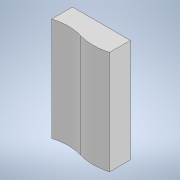
# Autodesk Inventor part: Ground2
Saved by Autodesk Inventor 2021 (Build 250183000, 183)
## iProperties
Created: 2022-07-02
Part Number: Ground2
Material: 一般
Document SubType Name: Modeling
Designer: tazak
Density: 1 g/cm^3
Appearance: 既定
Author: tazak
Autodesk Inventor part; units mm, degrees
ref_plane "YZ Plane" through (0, 0, 0) normal (1, 0, 0) x (0, 1, 0)
ref_plane "XZ Plane" through (0, 0, 0) normal (0, 1, 0) x (-1, 0, 0)
ref_plane "XY Plane" through (0, 0, 0) normal (0, 0, 1) x (1, 0, 0)
sketch "スケッチ1" plane through (0, 0, 0) normal (0, 0, 1) x (1, 0, 0)
  line L0 (2000, 2500) -> (4800, 2500)
  line L1 (4800, 2500) -> (4800, -2500)
  line L2 (4800, -2500) -> (2000, -2500)
  line L3 (2000, -2500) -> (2000, 2500)
  point P0 (0, 0)
  point P1 (2000, 0)
  dimension "d2" = 5000
  dimension "d5" = 2000
  dimension "d6" = 2800
  constraints: 8 end point, 2 parallel, 1 horizontal, 1 horizontal alignment, 1 midpoint, 1 perpendicular
  measures "d2" distance of L2.end L0.start
  measures "d5" distance from line of L3 point (0, 0)
  measures "d6" distance of L0.start L0.end
extrude "押し出し1" add sketch "スケッチ1" against normal blind 1000
sketch "スケッチ2" plane through (2000, -2500, 0) normal (0, -1, 0) x (1, 0, 0)
  circle A0 centre (700, 2400) radius 2500
  line L0 (0, 0) -> (2800, 0) projected
  point P0 (-2000, 0)
  point P1 (1400, 0)
  dimension "d7" = 5000
  constraints: 2 point on circle, 1 centre point, 1 midpoint
  measures "d7" diameter of A0
extrude "押し出し2" cut sketch "スケッチ2" against normal through all
sketch "スケッチ3" plane through (2000, -2500, -1000) normal (0, -1, 0) x (1, 0, 0)
  line L0 (2800, 1000) -> (1400, 1000) projected
  circle A0 centre (2100, -1400) radius 2500
  point P0 (-2000, 1000)
  dimension "d10" = 5000
  constraints: 2 point on circle, 1 centre point
  measures "d10" diameter of A0
extrude "押し出し3" add sketch "スケッチ3" against normal blind 5000 contours L0 A0 picked at (1910.2312, 1011.4384)
